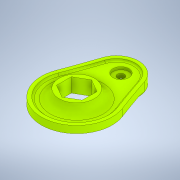
# Autodesk Inventor part: Follower
Saved by Autodesk Inventor 2021 (Build 250183000, 183)
## iProperties
Created: 2021-08-12
Part Number: Follower
Material: Generic
Document SubType Name: Modeling
Designer: Shammy Haider
Density: 1 g/cm^3
Appearance: Default
Author: Shammy Haider
Autodesk Inventor part; units mm, degrees
ref_plane "YZ Plane" through (0, 0, 0) normal (1, 0, 0) x (0, 1, 0)
ref_plane "XZ Plane" through (0, 0, 0) normal (0, 1, 0) x (-1, 0, 0)
ref_plane "XY Plane" through (0, 0, 0) normal (0, 0, 1) x (1, 0, 0)
sketch "Sketch1" plane through (0, 0, 0) normal (0, 1, 0) x (-1, 0, 0)
  circle A0 centre (0, 0) radius 40
  dimension "d0" = 80
  constraints: 1 centre point, 1 coincident
  measures "d0" diameter of A0
extrude "Extrusion1" add sketch "Sketch1" along normal mid plane 8
sketch "Sketch2" plane through (0, 4, 0) normal (0, 1, 0) x (1, 0, 0)
  circle A0 centre (0, 0) radius 40 projected
  circle A1 centre (0, 45) radius 25
  dimension "d3" = 50
  dimension "d4" = 45
  constraints: 1 centre point
  measures "d3" diameter of A1
  measures "d4" distance of A1.centre point (0, 0)
extrude "Extrusion2" add sketch "Sketch2" against normal blind 10 contours A1 A0 | A0 A1 picked at (-3.589, 33.1406) picked at (7.3164, 48.2743)
fillet "Fillet1" radius 1000 2 edges at (-22.1108, 0, -33.3333) (22.1108, 0, -33.3333)
fillet "Fillet2" radius 2 4 edges at (24.6822, -4, -48.9733) (-24.9136, -4, -42.9236) (0, -4, -20) (24.267, -4, -38.9905)
sketch "Sketch3" plane through (0, 4, 0) normal (0, 1, 0) x (1, 0, 0)
  arc A0 (-37.4315, 14.1026) -> (37.4315, 14.1026) centre (0, 0) ccw projected
  arc A1 (-37.4315, 14.1026) -> (-23.7371, 52.8455) centre (-973.2192, 366.6667) ccw projected
  arc A2 (23.7371, 52.8455) -> (-23.7371, 52.8455) centre (0, 45) ccw projected
  arc A3 (23.7371, 52.8455) -> (37.4315, 14.1026) centre (973.2192, 366.6667) ccw projected
  arc A4 (-33.6884, 12.6923) -> (33.6884, 12.6923) centre (0, 0) ccw
  arc A5 (-33.6884, 12.6923) -> (-19.9391, 51.5902) centre (-973.2192, 366.6667) ccw
  arc A6 (19.9391, 51.5902) -> (-19.9391, 51.5902) centre (0, 45) ccw
  arc A7 (19.9391, 51.5902) -> (33.6884, 12.6923) centre (973.2192, 366.6667) ccw
  dimension "d9" = 4
  constraints: 8 point on circle, 4 centre point, 3 other
  measures "d9" radial gap between concentric circles of A0 A4
extrude "Extrusion3" cut sketch "Sketch3" against normal blind 2 contours A5 A6 A7 A4
fillet "Fillet3" radius 2 4 edges at (0, 2, 36) (-26.6139, 2, -32.0706) (0, 2, -66) (26.6139, 2, -32.0706)
sketch "Sketch4" plane through (0, 2, 0) normal (0, 1, 0) x (1, 0, 0)
  line L0 (0, 16.7948) -> (14.5447, 8.3974)
  line L1 (14.5447, 8.3974) -> (14.5447, -8.3974)
  line L2 (14.5447, -8.3974) -> (0, -16.7948)
  line L3 (0, -16.7948) -> (-14.5447, -8.3974)
  line L4 (-14.5447, -8.3974) -> (-14.5447, 8.3974)
  line L5 (-14.5447, 8.3974) -> (0, 16.7948)
  point P0 (0, 0)
  point P1 (0, 0)
  constraints: 12 end point, 1 coincident, 13 other
extrude "Extrusion4" cut sketch "Sketch4" against normal through all
sketch "Sketch5" plane through (0, 2, 0) normal (0, 1, 0) x (1, 0, 0)
  circle A0 centre (0, 0) radius 20
  line L0 (0, -16.7948) -> (-14.5447, -8.3974) projected
  line L1 (-14.5447, -8.3974) -> (-14.5447, 8.3974) projected
  line L2 (-14.5447, 8.3974) -> (0, 16.7948) projected
  line L3 (0, 16.7948) -> (14.5447, 8.3974) projected
  line L4 (14.5447, 8.3974) -> (14.5447, -8.3974) projected
  line L5 (14.5447, -8.3974) -> (0, -16.7948) projected
  dimension "d17" = 40
  constraints: 1 centre point, 1 coincident
  measures "d17" diameter of A0
extrude "Extrusion5" add sketch "Sketch5" along normal blind 10
fillet "Fillet4" radius 10 1 edges at (-20, 2, 0)
sketch "Sketch6" plane through (0, 2, 0) normal (0, 1, 0) x (1, 0, 0)
  circle A0 centre (0, 50) radius 9
  circle A1 centre (0, 50) radius 4
  arc A2 (23.7371, 52.8455) -> (-23.7371, 52.8455) centre (0, 45) ccw projected
  point P0 (0, 0)
  dimension "d21" = 18
  dimension "d22" = 8
  dimension "d23" = 5
  constraints: 2 centre point, 1 coincident
  measures "d21" diameter of A0
  measures "d22" diameter of A1
  measures "d23" distance of A2.centre A0.centre
extrude "Extrusion6" cut sketch "Sketch6" against normal blind 3
extrude "Extrusion7" cut sketch "Sketch6" against normal through all contours A1
body "Solid1"
